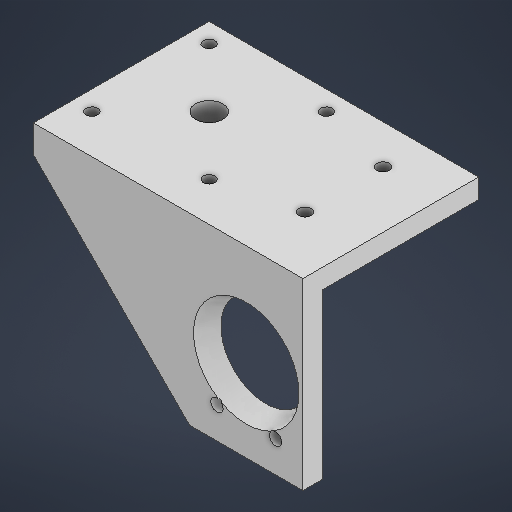
# Autodesk Inventor part: Tensioner Top
Saved by Autodesk Inventor 2025.1 (Build 291241000, 241)
## iProperties
Created: 2025-02-02
Part Number: Tensioner Top
Material: Generic
Document SubType Name: Modeling
Designer: jerem
Density: 1 g/cm^3
Appearance: Default
Author: jerem
## iProperties of the stored document Tensioner Top_3DPrint.ipt
Created: 2025-02-02
Part Number: Tensioner Top_3DPrint
Material: Generic
Document SubType Name: Modeling
Designer: jerem
Density: 1 g/cm^3
Appearance: Default
Author: jerem
Autodesk Inventor part; units mm, degrees
ref_plane "YZ Plane" through (0, 0, 0) normal (1, 0, 0) x (0, 1, 0)
ref_plane "XZ Plane" through (0, 0, 0) normal (0, 1, 0) x (-1, 0, 0)
ref_plane "XY Plane" through (0, 0, 0) normal (0, 0, 1) x (1, 0, 0)
sketch "Sketch1" plane through (0, 0, 0) normal (0, 1, 0) x (-1, 0, 0)
  line L0 (-20, 20) -> (20, 20)
  line L1 (20, 20) -> (20, -20)
  line L2 (20, -20) -> (-20, -20)
  line L3 (-20, -20) -> (-20, 20)
  line L4 (-20, 20) -> (20, -20) construction
  line L5 (20, 20) -> (-20, -20) construction
  circle A0 centre (15, -15) radius 1.5
  circle A1 centre (-15, -15) radius 1.5
  circle A2 centre (-15, 15) radius 1.5
  circle A3 centre (15, 15) radius 1.5
  line L6 (15, 15) -> (15, -15) construction
  line L7 (-15, -15) -> (15, -15) construction
  line L8 (-15, -15) -> (-15, 15) construction
  line L9 (-20, 20) -> (-49, 20)
  line L10 (-49, 20) -> (-49, -20)
  line L11 (-49, -20) -> (-20, -20)
  circle A4 centre (0, 0) radius 3.5
  line L12 (20, 20) -> (20, 25)
  line L13 (20, 25) -> (-49, 25)
  line L14 (-49, 25) -> (-49, 20)
  line L15 (-34.5, -20) -> (-34.5, -10) construction
  line L16 (-34.5, -10) -> (-34.5, 10) construction
  circle A5 centre (-34.5, -10) radius 1.6
  circle A6 centre (-34.5, 10) radius 1.6
  dimension "d0" = 40
  dimension "d1" = 40
  dimension "d2" = 30
  dimension "d3" = 3
  dimension "d26" = 7
  dimension "d27" = 29
  dimension "d29" = 5
  dimension "d40" = 10
  dimension "d41" = 20
  dimension "d42" = 3.2
  constraints: 34 end point, 8 perpendicular, 7 centre point, 5 point on line, 4 equal radius, 3 coincident, 3 midpoint, 3 parallel, 2 horizontal, 2 vertical
  measures "d0" distance of L1.end L2.end
  measures "d1" distance of L0.end L1.end
  measures "d2" distance of L7.start L6.end
  measures "d3" diameter of A0
  measures "d26" diameter of A4
  measures "d27" distance between parallel lines of L10 L3
  measures "d29" distance between parallel lines of L0 L13
  measures "d40" distance of L15.start L15.end
  measures "d41" distance of L15.end L16.end
  measures "d42" diameter of A5
extrude "Extrusion1" add sketch "Sketch1" along normal blind 5
extrude "Extrusion4" add sketch "Sketch1" against normal blind 42 contours L9 L14 L13 L12 L0
sketch "Sketch2" plane through (-20, 5, 25) normal (0, 0, 1) x (1, 0, 0)
  line L0 (69, -47) -> (69, 0) projected
  line L1 (0, 0) -> (69, 0) projected
  line L2 (0, -47) -> (0, 0) projected
  line L3 (69, -47) -> (0, -47) projected
  line L4 (69, -47) -> (40, -47)
  line L5 (40, -47) -> (40, 0)
  line L6 (40, 0) -> (69, 0)
  line L7 (69, 0) -> (69, -47)
  circle A0 centre (54.5, -26) radius 11.5
  line L8 (54.5, -26) -> (54.5, -47) construction
  line L9 (69, -47) -> (0, -47) projected
  line L10 (43, -32.6395) -> (43, -19.3605)
  line L11 (43, -19.3605) -> (54.5, -12.7209)
  line L12 (54.5, -12.7209) -> (66, -19.3605)
  line L13 (66, -19.3605) -> (66, -32.6395)
  line L14 (66, -32.6395) -> (54.5, -39.2791)
  line L15 (54.5, -39.2791) -> (43, -32.6395)
  line L16 (54.5, -39) -> (62, -39) construction
  line L17 (54.5, -39) -> (47, -39) construction
  circle A1 centre (62, -39) radius 1.6
  circle A2 centre (47, -39) radius 1.6
  point P0 (20, -5)
  point P1 (54.5, -26)
  point P2 (48.75, -35.9593)
  point P3 (60.25, -35.9593)
  point P4 (43, -26)
  point P5 (66, -26)
  point P6 (60.25, -16.0407)
  point P7 (48.75, -16.0407)
  dimension "d32" = 29
  dimension "d33" = 21
  dimension "d34" = 23
  dimension "d37" = 3.2
  dimension "d39" = 8
  dimension "d46" = 15
  constraints: 26 end point, 5 point on line, 3 centre point, 3 tangent, 2 coincident, 2 horizontal, 2 parallel, 2 perpendicular, 1 collinear, 1 equal radius, 1 midpoint, 1 vertical, 13 other
  measures "d32" distance between parallel lines of L0 L5
  measures "d33" distance of L8.start L8.end
  measures "d34" diameter of A0
  measures "d37" diameter of A2
  measures "d39" distance between parallel lines of L4 L17
  measures "d46" distance of L16.end A2.centre
extrude "Extrusion5" cut sketch "Sketch2" against normal up to surface (5 mm away) contours A0 | A1 | A2
chamfer "Chamfer4" distance 40 angle 45 1 edges at (-20, -42, 22.5)
chamfer "Chamfer5" distance 2 distance2 5 1 edges at (23, -21, 25) measured on face at (22.5, -21, 25)
body "Solid1"
